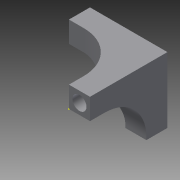
# Autodesk Inventor part: Crossbar holder
Saved by Autodesk Inventor 2015 (Build 190159000, 159)
## iProperties
Created: 2014-11-01
Part Number: Crossbar holder
Material: Generic
Document SubType Name: Modeling
Designer: Scott
Density: 1 g/cm^3
Appearance: Default
Author: Scott
Autodesk Inventor part; units mm, degrees
ref_plane "YZ Plane" through (0, 0, 0) normal (1, 0, 0) x (0, 1, 0)
ref_plane "XZ Plane" through (0, 0, 0) normal (0, 1, 0) x (-1, 0, 0)
ref_plane "XY Plane" through (0, 0, 0) normal (0, 0, 1) x (1, 0, 0)
sketch "Sketch1" plane through (0, 0, 0) normal (0, 1, 0) x (-1, 0, 0)
  point P0 (0, 0)
sketch "Sketch2" plane through (0, 0, 0) normal (0, 1, 0) x (-1, 0, 0)
  line L0 (0, 0) -> (-12, 0)
  line L1 (-12, 0) -> (-12, -38.1)
  line L2 (-12, -38.1) -> (-12, -44.1)
  line L3 (-12, -44.1) -> (-6, -44.1)
  line L4 (-6, -44.1) -> (32.1, -44.1)
  line L5 (32.1, -44.1) -> (32.1, -32.1)
  line L6 (32.1, -32.1) -> (0, -32.1)
  line L7 (0, -32.1) -> (0, 0)
  dimension "d0" = 12
  dimension "d1" = 38.1
  dimension "d2" = 6
  dimension "d3" = 6
  dimension "d4" = 38.1
  dimension "d5" = 12
  constraints: 16 end point, 5 perpendicular, 2 point on line, 1 horizontal
  measures "d0" distance of L0.start L0.end
  measures "d1" distance of L0.end L1.end
  measures "d2" distance of L1.end L2.end
  measures "d3" distance of L2.end L3.end
  measures "d4" distance of L3.end L4.end
  measures "d5" distance of L4.end L5.end
extrude "Extrusion1" add sketch "Sketch2" along normal blind 12
sketch "Sketch3" plane through (0, 0, 0) normal (0, 0, 1) x (1, 0, 0)
  point P0 (0, 0)
sketch "Sketch4" plane through (0, 0, 0) normal (0, 0, 1) x (1, 0, 0)
  line L0 (0, 0) -> (0, 12)
  line L1 (0, 12) -> (12, 12)
  circle A0 centre (6, 6) radius 4
  dimension "d8" = 8
  constraints: 4 end point, 1 centre point, 1 perpendicular, 1 vertical
  measures "d8" diameter of A0
extrude "Extrusion2" cut sketch "Sketch4" against normal blind 12.7
sketch "Sketch5" plane through (-32.1, 0, -44.1) normal (-1, 0, 0) x (0, 0, 1)
  line L0 (0, 12) -> (0, 0)
  line L1 (0, 0) -> (12, 0)
  line L2 (12, 0) -> (12, 12) projected
  circle A0 centre (6, 6) radius 4
  point P0 (44.1, 0)
  dimension "d11" = 8
  constraints: 4 end point, 1 centre point, 1 perpendicular, 1 vertical
  measures "d11" diameter of A0
extrude "Extrusion3" cut sketch "Sketch5" against normal blind 12.7
sketch "Sketch6" plane through (0, 0, 0) normal (0, -1, 0) x (1, 0, 0)
  line L0 (0, -32.1) -> (12, -32.1)
  line L1 (12, 0) -> (12, -44.1) projected
  line L2 (-32.1, -32.1) -> (0, -32.1) projected
  line L3 (0, -32.1) -> (0, -44.1)
  line L4 (12, -32.1) -> (12, -44.1)
  line L5 (12, -44.1) -> (0, -44.1)
  point P0 (0, 0)
  constraints: 8 end point, 2 collinear, 1 perpendicular, 1 point on line, 1 vertical
extrude "Extrusion4" add sketch "Sketch6" along normal blind 25.4
fillet "Fillet1" radius 23.8125 2 edges at (0, 0, -38.1) (6, 0, -32.1)
fillet "Fillet2" radius 23.8125 1 edges at (0, -5.9062, -32.1)
sketch "Sketch7" plane through (0, -25.4, 0) normal (0, -1, 0) x (1, 0, 0)
  line L0 (12, -44.1) -> (12, -32.1)
  line L1 (12, -32.1) -> (0, -32.1)
  line L2 (0, -32.1) -> (12, -32.1) projected
  circle A0 centre (6, -38.1) radius 3
  point P0 (0, 0)
  dimension "d18" = 6
  constraints: 4 end point, 1 centre point, 1 collinear, 1 vertical
  measures "d18" diameter of A0
extrude "Extrusion5" cut sketch "Sketch7" against normal blind 12.7
body "Solid1"
